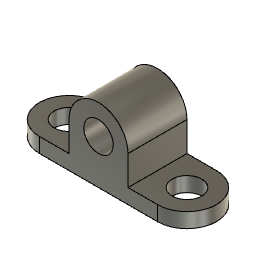
Figure A4 v2 (Autodesk Fusion 360 design; units mm, degrees)
Autodesk Fusion 360 part; units mm, degrees
note: some values were not read from the file. Set by a fixed rule: which sketch regions a step uses.
sketch "Sketch4" plane through (0, 0, 0) normal (0, 0, 1) x (1, 0, 0)
  line L0 (40, 20) -> (-40, 20)
  line L1 (-40, 20) -> (-40, -20)
  line L2 (-40, -20) -> (40, -20)
  line L3 (40, -20) -> (40, 20)
  line L4 (40, 20) -> (-40, -20) construction
  line L5 (-40, 20) -> (40, -20) construction
  line L6 (20, 20) -> (20, -20) construction
  circle A0 centre (40, 0) radius 20
  circle A1 centre (-40, 0) radius 20
  circle A2 centre (-40, 0) radius 10
  circle A3 centre (40, 0) radius 10
  line L7 (-20, 20) -> (-20, 10) construction
  line L8 (-20, 0) -> (-20, -20) construction
  dimension "d11" = 80
  dimension "d12" = 40
  dimension "d13" = 40
  dimension "d14" = 20
  dimension "d15" = 40
  dimension "d16" = 40
  dimension "d17" = 20
  dimension "d18" = 20
  constraint horizontal L0
  constraint perpendicular L0 L1
  constraint parallel L0 L2
  constraint parallel L1 L3
  constraint coincident L4 origin
  constraint coincident L5 origin
  constraint coincident L0 L7.start
  constraint coincident L2 L8.end
  constraint perpendicular L2 L7
  constraint coincident L0 L6.start
  constraint coincident L2 L6.end
  constraint perpendicular L2 L6
  constraint midpoint L3 A0.centre
  constraint midpoint L1 A1.centre
  constraint concentric A1 A2
  constraint concentric A0 A3
  constraint coincident L5 L7.end
  constraint coincident A1 L8.start
  constraint collinear L7 L8
  measures "d11" distance of L1.end L2.end
  measures "d12" distance of L0.end L1.end
  measures "d13" distance of L6 L7
  measures "d14" distance of L3 L6
  measures "d15" diameter of A0
  measures "d16" diameter of A1
  measures "d17" diameter of A2
  measures "d18" diameter of A3
extrude "Extrude2" add sketch "Sketch4" along normal blind 10 contours L0 L2 A0 A1 | L3 A0 A3 | L3 A0 A3 | L1 A1 A2 | L1 A1 A2
sketch "Sketch5" plane through (0, 0, 0) normal (0, 1, 0) x (1, 0, 0)
  line L0 (-20, 0) -> (20, 0)
  line L1 (20, 0) -> (20, -30)
  line L2 (-20, -30) -> (-20, 0)
  line L3 (-40, 0) -> (-40, -10)
  circle A0 centre (0, -30) radius 10
  arc A1 (-20, -30) -> (20, -30) centre (0, -30) ccw
  dimension "d21" = 40
  dimension "d22" = 30
  dimension "d23" = 20
  constraint horizontal L0
  constraint vertical L1
  constraint vertical L2
  constraint concentric A0 A1
  measures "d21" distance of L0.start L0.end
  measures "d22" distance of L0.start L2.start
  measures "d23" distance of L2 L3
extrude "Extrude3" add sketch "Sketch5" along normal mid plane 40
sketch "Sketch1" plane through (0, 0, 0) normal (0, 0, 1) x (1, 0, 0)
  line L0 (40, 20) -> (-40, 20)
  line L1 (-40, 20) -> (-40, -20)
  line L2 (-40, -20) -> (40, -20)
  line L3 (40, -20) -> (40, 20)
  line L4 (40, 20) -> (-40, -20) construction
  line L5 (-40, 20) -> (40, -20) construction
  circle A0 centre (-40, 0) radius 20
  circle A1 centre (40, 0) radius 20
  circle A2 centre (-40, 0) radius 10
  circle A3 centre (40, 0) radius 10
  dimension "d1" = 80
  dimension "d2" = 40
  dimension "d3" = 40
  dimension "d4" = 40
  dimension "d5" = 20
  dimension "d6" = 20
  constraint horizontal L0
  constraint perpendicular L0 L1
  constraint parallel L0 L2
  constraint parallel L1 L3
  constraint coincident L4 origin
  constraint coincident L5 origin
  constraint midpoint L1 A0.centre
  constraint midpoint L3 A1.centre
  constraint concentric A0 A2
  constraint concentric A1 A3
  measures "d1" distance of L1.end L2.end
  measures "d2" distance of L0.end L1.end
  measures "d3" diameter of A0
  measures "d4" diameter of A1
  measures "d5" diameter of A2
  measures "d6" diameter of A3
extrude "Extrude1" [suppressed]
sketch "Sketch3" plane through (0, 0, 10) normal (0, 0, 1) x (-1, 0, 0)
  circle A0 centre (40, 0) radius 10
  circle A1 centre (-40, 0) radius 10
  arc A2 (-40, 20) -> (-40, -20) centre (-40, 0) ccw
  line L0 (-40, -20) -> (40, -20)
  arc A3 (40, -20) -> (40, 20) centre (40, 0) ccw
  line L1 (40, 20) -> (-40, 20)
named bodies: "Main Part"
